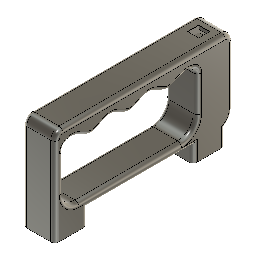
main_handle (Autodesk Fusion 360 design; units mm, degrees)
Autodesk Fusion 360 part; units mm, degrees
sketch "Skizze1" plane through (0, 0, 0) normal (1, 0, 0) x (0, 1, 0)
  line L0 (0, 0) -> (0, 60)
  line L1 (0, 60) -> (111.25, 60)
  line L2 (111.25, 60) -> (111.25, 10)
  line L3 (111.25, 10) -> (106.25, 10)
  line L4 (106.25, 10) -> (106.25, 0)
  line L5 (106.25, 0) -> (86.25, 0)
  line L6 (86.25, 0) -> (86.25, 10)
  line L7 (86.25, 10) -> (20, 10)
  line L8 (20, 10) -> (20, 0)
  line L9 (20, 0) -> (0, 0)
  dimension "d1" = 20
  dimension "d2" = 20
  dimension "d3" = 86.25
  dimension "d4" = 5
  dimension "d5" = 60
  dimension "d6" = 10
  dimension "d7" = 10
  constraint coincident L0.start L9.end
  constraint vertical L0
  constraint perpendicular L0 L1
  constraint perpendicular L1 L2
  constraint perpendicular L2 L3
  constraint perpendicular L3 L4
  constraint perpendicular L4 L5
  constraint perpendicular L3 L6
  constraint perpendicular L6 L7
  constraint perpendicular L3 L8
  constraint perpendicular L0 L9
  constraint collinear L5 L9
  measures "d1" distance of L8.end L0.start
  measures "d2" distance of L4.end L5.end
  measures "d3" distance of L0 L6
  measures "d4" distance of L2.end L3.end
  measures "d5" distance of L0.start L0.end
  measures "d6" distance of L7.end L8.end
  measures "d7" distance of L3.end L4.end
extrude "Extrusion1" add sketch "Skizze1" along normal mid plane 20
sketch "Skizze2" plane through (10, 0, 0) normal (1, 0, 0) x (0, 1, 0)
  line L0 (20, 0) -> (20, 10)
  line L1 (20, 10) -> (86.25, 10)
  line L2 (86.25, 10) -> (86.25, 0)
  line L3 (86.25, 0) -> (106.25, 0)
  line L4 (106.25, 0) -> (106.25, 10)
  line L5 (106.25, 10) -> (111.25, 10)
  line L6 (111.25, 10) -> (111.25, 60)
  line L7 (111.25, 60) -> (0, 60)
  line L8 (0, 60) -> (0, 0)
  line L9 (0, 0) -> (20, 0)
  spline S0 degree 5 poles (5, 50) (5.24, 50.1771) (5.72, 50.5116) (6.44, 50.9545) (7.4, 51.4271) (8.6, 51.8223) (9.8, 52.0253) (11, 52.0432) (12.2, 51.888) (13.4, 51.5778) (14.6, 51.1376) (15.8, 50.5994) (17, 50.0027) (18.2, 49.395) (19.4, 48.8323) (20.6, 48.3716) (21.8, 48.0643) (23, 47.9481) (24.2, 48.0405) (25.4, 48.3314) (26.6, 48.7887) (27.8, 49.3644) (29, 50.0005) (30.2, 50.6345) (31.4, 51.2058) (32.6, 51.6596) (33.8, 51.9511) (35, 52.0506) (36.2, 51.9469) (37.4, 51.6524) (38.6, 51.1981) (39.8, 50.6291) (41, 50.0001) (42.2, 49.3707) (43.4, 48.8008) (44.6, 48.3457) (45.8, 48.0513) (47, 47.9491) (48.2, 48.0513) (49.4, 48.3457) (50.6, 48.8008) (51.8, 49.3707) (53, 50.0001) (54.2, 50.6291) (55.4, 51.1981) (56.6, 51.6524) (57.8, 51.9469) (59, 52.0506) (60.2, 51.9511) (61.4, 51.6596) (62.6, 51.2058) (63.8, 50.6345) (65, 50.0005) (66.2, 49.3644) (67.4, 48.7887) (68.6, 48.3314) (69.8, 48.0405) (71, 47.9481) (72.2, 48.0643) (73.4, 48.3716) (74.6, 48.8323) (75.8, 49.395) (77, 50.0027) (78.2, 50.5994) (79.4, 51.1376) (80.6, 51.5778) (81.8, 51.888) (83, 52.0432) (84.2, 52.0253) (85.4, 51.8223) (86.6, 51.4271) (87.56, 50.9545) (88.28, 50.5116) (88.76, 50.1771) (89, 50) knots 0 0 0 0 0 0 0.01428571 0.02857143 0.04285714 0.05714286 0.07142857 0.08571429 0.1 0.11428571 0.12857143 0.14285714 0.15714286 0.17142857 0.18571429 0.2 0.21428571 0.22857143 0.24285714 0.25714286 0.27142857 0.28571429 0.3 0.31428571 0.32857143 0.34285714 0.35714286 0.37142857 0.38571429 0.4 0.41428571 0.42857143 0.44285714 0.45714286 0.47142857 0.48571429 0.5 0.51428571 0.52857143 0.54285714 0.55714286 0.57142857 0.58571429 0.6 0.61428571 0.62857143 0.64285714 0.65714286 0.67142857 0.68571429 0.7 0.71428571 0.72857143 0.74285714 0.75714286 0.77142857 0.78571429 0.8 0.81428571 0.82857143 0.84285714 0.85714286 0.87142857 0.88571429 0.9 0.91428571 0.92857143 0.94285714 0.95714286 0.97142857 0.98571429 1 1 1 1 1 1
  line L10 (5, 50) -> (89, 50)
  line L11 (5, 50) -> (5, 15)
  line L12 (5, 15) -> (89, 15)
  line L13 (89, 15) -> (89, 50)
  point P0 (11, 52)
  point P1 (17, 50)
  point P2 (23, 48)
  point P3 (29, 50)
  point P4 (35, 52)
  point P5 (41, 50)
  point P6 (47, 48)
  point P7 (53, 50)
  point P8 (59, 52)
  point P9 (65, 50)
  point P10 (71, 48)
  point P11 (77, 50)
  point P12 (83, 52)
  dimension "d10" = 5
  dimension "d11" = 6
  dimension "d12" = 6
  dimension "d13" = 6
  dimension "d14" = 6
  dimension "d15" = 6
  dimension "d16" = 6
  dimension "d17" = 6
  dimension "d18" = 6
  dimension "d19" = 6
  dimension "d20" = 6
  dimension "d21" = 6
  dimension "d22" = 6
  dimension "d24" = 10
  dimension "d25" = 10
  dimension "d26" = 6
  dimension "d27" = 6
  dimension "d28" = 2
  dimension "d29" = 2
  dimension "d30" = 2
  dimension "d31" = 2
  dimension "d32" = 2
  dimension "d33" = 2
  dimension "d34" = 2
  dimension "d35" = 35
  constraint coincident P1 L10
  constraint coincident P3 L10
  constraint coincident P5 L10
  constraint coincident P7 L10
  constraint coincident P9 L10
  constraint coincident P11 L10
  constraint perpendicular L10 L11
  constraint perpendicular L11 L12
  constraint perpendicular L10 L13
  measures "d10" distance of L8 S0.start
  measures "d11" distance of S0.start P0
  measures "d12" horizontal distance of P0 P1
  measures "d13" horizontal distance of P1 P2
  measures "d14" horizontal distance of P2 P3
  measures "d15" horizontal distance of P3 P4
  measures "d16" horizontal distance of P4 P5
  measures "d17" horizontal distance of P5 P6
  measures "d18" horizontal distance of P6 P7
  measures "d19" horizontal distance of P7 P8
  measures "d20" horizontal distance of P8 P9
  measures "d21" horizontal distance of P9 P10
  measures "d22" horizontal distance of P10 P11
  measures "d24" distance of L7 S0.end
  measures "d25" distance of L7 S0.start
  measures "d26" horizontal distance of P11 P12
  measures "d27" distance of S0.end P12
  measures "d28" distance of L10 P12
  measures "d29" distance of P10 L10
  measures "d30" distance of P8 L10
  measures "d31" distance of P6 L10
  measures "d32" distance of P4 L10
  measures "d33" distance of P2 L10
  measures "d34" distance of P0 L10
  measures "d35" distance of S0.start L11.end
extrude "Extrusion2" cut sketch "Skizze2" against normal through all contours S0 L10 | S0 L10 L11 L12 L13 | S0 L10 | S0 L10 | S0 L10 picked at (12.3798, 50.2951) picked at (36.4294, 50.2871) picked at (82.08, 50.476) picked at (60.4482, 50.2803)
fillet "Abrundung11" radius 10 3 edges at (0, 89, 15) (0, 111.25, 10) (0, 5, 15)
fillet "Abrundung12" radius 5 2 edges at (0, 111.25, 60) (0, 0, 60)
fillet "Abrundung13" radius 5 2 edges at (0, 89, 50) (0, 5, 50)
fillet "Abrundung14" radius 2.5 28 edges at (-10, 0, 27.5) (-10, 1.4645, 58.5355) (-10, 55.625, 60) (-10, 109.7855, 58.5355) (-10, 111.25, 36.8301) (-10, 109.9103, 13.6603) (-10, 6.1556, 50.1612) (-10, 47, 48) (-10, 87.8413, 50.1649) (-10, 89, 35.9821) (-10, 86.0711, 17.9289) (-10, 47, 15) (-10, 7.9289, 17.9289) (-10, 5, 35.9821) (10, 7.9289, 17.9289) (10, 47, 15) (10, 86.0711, 17.9289) (10, 89, 35.9821) (10, 87.8444, 50.1612) (10, 47, 48) (10, 6.1587, 50.1649) (10, 5, 35.9821) (10, 109.9103, 13.6603) (10, 111.25, 36.8301) (10, 109.7855, 58.5355) (10, 55.625, 60) (10, 1.4645, 58.5355) (10, 0, 27.5)
fillet "Abrundung15" radius 2.5 2 edges at (-10, 53.125, 10) (10, 53.125, 10)
fillet "Abrundung16" radius 2.5 6 edges at (-10, 86.25, 6.25) (10, 86.25, 6.25) (10, 106.25, 6.535) (-10, 106.25, 6.535) (-10, 20, 6.25) (10, 20, 6.25)
sketch "Skizze3" plane through (0, 0, 0) normal (0, 0, -1) x (1, 0, 0)
  arc A0 (-10, -103.75) -> (-7.5, -106.25) centre (-7.5, -103.75) ccw
  line L0 (-7.5, -106.25) -> (7.5, -106.25)
  arc A1 (7.5, -106.25) -> (10, -103.75) centre (7.5, -103.75) ccw
  line L1 (10, -103.75) -> (10, -88.75)
  arc A2 (10, -88.75) -> (7.5, -86.25) centre (7.5, -88.75) ccw
  line L2 (7.5, -86.25) -> (-7.5, -86.25)
  arc A3 (-7.5, -86.25) -> (-10, -88.75) centre (-7.5, -88.75) ccw
  line L3 (-10, -88.75) -> (-10, -103.75)
  line L4 (0, -1.75) -> (0, -22.5)
  point P0 (0, -96.25)
  point P1 (0, -10)
  dimension "d69" = 86.25
  dimension "d70" = 10
  constraint coincident P1 L4
  constraint coincident P0 L4
  measures "d69" distance of P0 P1
  measures "d70" distance of L0 P0
hole "Bohrung1" at (0, 96.25, 0) at (0, 10, 0) direction (0, 0, 1) diameter 3.2 depth 15 tip angle 180
ref_plane "Arbeitsebene1" through (0, 10, 40) normal (0, 0, -1) x (0, 1, 0)
sketch "Skizze5" plane through (0, 0, 60) normal (0, 0, 1) x (-1, 0, 0)
  line L0 (7.5, -5) -> (-7.5, -5)
  line L1 (-7.5, -5) -> (-7.5, -106.25)
  line L2 (-7.5, -106.25) -> (7.5, -106.25)
  line L3 (7.5, -106.25) -> (7.5, -5)
  line L4 (3.5, -103.25) -> (-3.5, -103.25)
  line L5 (-3.5, -103.25) -> (-3.5, -96.25)
  line L6 (-3.5, -96.25) -> (3.5, -96.25)
  line L7 (3.5, -96.25) -> (3.5, -103.25)
  line L8 (0, -1.75) -> (0, -22.5)
  dimension "d82" = 7
  dimension "d83" = 7
  dimension "d84" = 3
  dimension "d85" = 3.5
  constraint horizontal L4
  constraint vertical L5
  constraint horizontal L6
  constraint vertical L7
  measures "d82" distance of L5.end L6.end
  measures "d83" distance of L4.end L5.end
  measures "d84" distance of L2 L4
  measures "d85" distance of L5 L8
extrude "Extrusion4" cut sketch "Skizze5" against normal blind 4 contours L4 L5 L6 L7
sketch "Skizze7" plane through (-3.5, 0, 0) normal (1, 0, 0) x (0, 1, 0)
  line L0 (103.25, 60) -> (96.25, 60)
  line L1 (96.25, 60) -> (96.25, 56)
  line L2 (96.25, 56) -> (103.25, 56)
  line L3 (103.25, 56) -> (103.25, 60)
  line L4 (103.25, 56) -> (103.25, 28.7053)
  line L5 (103.25, 28.7053) -> (100.25, 20.4629)
  line L6 (104.25, 19.7576) -> (107.25, 28)
  line L7 (107.25, 28) -> (107.25, 58)
  line L8 (107.25, 58) -> (103.25, 58)
  line L9 (103.25, 58) -> (103.25, 56)
  line L10 (100.25, 20.4629) -> (100.25, -0.2424)
  line L11 (104.25, -0.2424) -> (100.25, -0.2424)
  line L12 (104.25, 19.7576) -> (104.25, -0.2424)
  dimension "d92" = 4
  dimension "d93" = 4
  dimension "d94" = 160
  dimension "d95" = 30
  dimension "d125" = 20
  dimension "d126" = 4
  dimension "d127" = 3
  constraint coincident L2.end L3.start
  constraint perpendicular L2 L4
  constraint perpendicular L2 L7
  constraint midpoint L3 L8.end
  constraint perpendicular L3 L8
  constraint parallel L5 L6
  constraint vertical L10
  constraint parallel L10 L12
  constraint perpendicular L10 L11
  measures "d92" distance of L5 L6
  measures "d93" distance of L4 L7
  measures "d94" angle of L4 L5
  measures "d95" distance of L6.end L7.end
  measures "d125" distance of L6.start L11
  measures "d126" distance of L10 L12
  measures "d127" horizontal distance of L4.end L5.end
extrude "Extrusion6" cut sketch "Skizze7" along normal blind 7 contours L3 L4 L5 L6 L7 L8 L9 L10 L11 L12
ref_plane "Arbeitsebene2" through (0, 96.25, 5) normal (0, 0, -1) x (0, 1, 0)
sketch "Skizze12" plane through (0, 96.25, 5) normal (0, 0, -1) x (1, 0, 0)
  line L0 (3, 90) -> (-3, 90)
  line L1 (-3, 90) -> (-3, -3.75)
  line L2 (-3, -3.75) -> (3, -3.75)
  line L3 (3, -3.75) -> (3, 90)
  point P0 (-1.6, 86.25)
  dimension "d119" = 6
  dimension "d120" = 3.75
  dimension "d121" = 3
  dimension "d122" = 3.75
  constraint horizontal L0
  constraint vertical L1
  constraint horizontal L2
  constraint vertical L3
  measures "d119" distance of L1.end L2.end
  measures "d120" distance of origin L2
  measures "d121" distance of origin L3
  measures "d122" vertical distance of L0.end P0
extrude "Extrusion10" cut sketch "Skizze12" against normal blind 3
equation "d11 = fingerdist"
equation "d12 = fingerdist"
equation "d13 = fingerdist"
equation "d14 = fingerdist"
equation "d15 = fingerdist"
equation "d16 = fingerdist"
equation "d17 = fingerdist"
equation "d18 = fingerdist"
equation "d19 = fingerdist"
equation "d20 = fingerdist"
equation "d21 = fingerdist"
equation "d22 = fingerdist"
equation "d26 = fingerdist"
equation "d27 = fingerdist"
equation "fingerdist = 6 mm"
equation "d120 = ( 7.5 / 2 ) * 1 mm"
equation "d122 = ( 7.5 / 2 ) * 1 mm"
